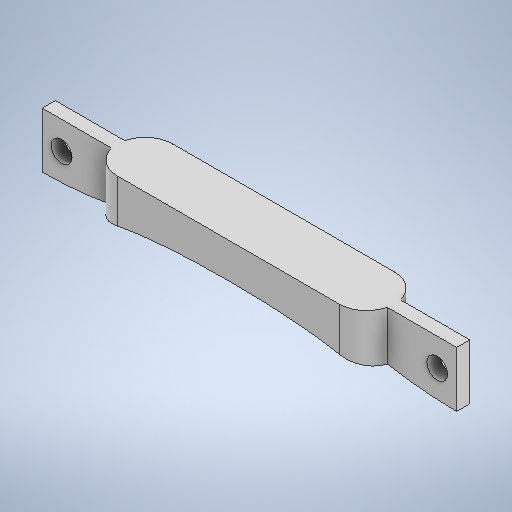
# Autodesk Inventor part: AllFretBars
Saved by Autodesk Inventor 2025.1 (Build 291241000, 241)
## iProperties
Created: 2025-11-05
Part Number: AllFretBars
Material: Generic
Document SubType Name: Modeling
Designer: Juxin
Density: 1 g/cm^3
Appearance: Default
Author: Juxin
Autodesk Inventor part; units mm, degrees
ref_plane "YZ Plane" through (0, 0, 0) normal (1, 0, 0) x (0, 1, 0)
ref_plane "XZ Plane" through (0, 0, 0) normal (0, 1, 0) x (-1, 0, 0)
ref_plane "XY Plane" through (0, 0, 0) normal (0, 0, 1) x (1, 0, 0)
sketch "Sketch1" plane through (0, 0, 0) normal (0, 1, 0) x (-1, 0, 0)
  line L0 (77.4625, -7.85) -> (77.4625, -4.85)
  line L1 (0, 0) -> (17.4625, 0) construction
  line L2 (77.4625, -6.35) -> (77.4625, -4.85)
  line L3 (77.4625, -4.85) -> (61.5875, -4.85)
  line L4 (61.5875, -7.85) -> (77.4625, -7.85)
  line L5 (61.5875, -4.85) -> (61.5875, 0)
  line L6 (61.5875, -7.85) -> (61.5875, -12.7)
  line L7 (61.5875, 0) -> (30, 0)
  line L8 (61.5875, -12.7) -> (30, -12.7)
  line L9 (-17.4625, -7.85) -> (-17.4625, -4.85)
  line L10 (-17.4625, -6.35) -> (-17.4625, -4.85)
  line L11 (-17.4625, -4.85) -> (-1.5875, -4.85)
  line L12 (-1.5875, -7.85) -> (-17.4625, -7.85)
  line L13 (-1.5875, -4.85) -> (-1.5875, 0)
  line L14 (-1.5875, -7.85) -> (-1.5875, -12.7)
  line L15 (-1.5875, 0) -> (30, 0)
  line L16 (-1.5875, -12.7) -> (30, -12.7)
  dimension "d23" = 1.5
  dimension "d24" = 15.875
  dimension "d25" = 3
  dimension "d27" = 63.175
  dimension "d117" = 12.7
  constraints: 34 end point, 2 horizontal, 2 midpoint, 2 perpendicular, 2 point on line
  measures "d23" distance of L0.end L2.start
  measures "d24" distance of L0.end L3.end
  measures "d25" distance of L3.end L4.start
  measures "d27" distance of L13.end L5.end
  measures "d117" distance of L6.end L5.end
extrude "Extrusion1" add sketch "Sketch1" along normal blind 12.7
sketch "Sketch3" plane through (1.5875, 0, -12.7) normal (0, 0, -1) x (-1, 0, 0)
  line L0 (0, 0) -> (63.175, 0) projected
  ellipse E0 centre (31.5875, 0) end of major axis (31.5875, 4.6466) minor radius 31.5875
  point P0 (1.5875, 0)
  constraints: 1 horizontal alignment, 1 midpoint, 2 other
extrude "Extrusion15" cut sketch "Sketch3" against normal blind 20.6375
sketch "Sketch4" plane through (-77.4625, 12.7, -4.85) normal (0, 0, 1) x (1, 0, 0)
  line L0 (15.875, -12.7) -> (15.875, 0) projected
  line L1 (15.875, -6.35) -> (4.445, -6.35)
  circle A0 centre (4.445, -6.35) radius 2.3876
  line L2 (79.05, -12.7) -> (79.05, 0) projected
  line L3 (79.05, -6.35) -> (90.48, -6.35)
  circle A1 centre (90.48, -6.35) radius 2.3876
  point P0 (77.4625, -12.7)
  dimension "d111" = 11.43
  dimension "d112" = 4.7752
  dimension "d113" = 11.43
  dimension "d114" = 4.7752
  constraints: 4 end point, 2 centre point, 2 coincident, 2 horizontal, 2 midpoint
  measures "d111" distance of L1.start L1.end
  measures "d112" diameter of A0
  measures "d113" distance of L3.start L3.end
  measures "d114" diameter of A1
extrude "Extrusion16" cut sketch "Sketch4" against normal blind 58.7375
fillet "Fillet1" radius 92.075 2 edges at (1.5875, 0, -6.35) (-61.5875, 0, -6.35)
fillet "Fillet2" radius 6.35 4 edges at (1.5875, 7.0818, -12.7) (-61.5875, 7.0818, -12.7) (-61.5875, 7.0818, 0) (1.5875, 7.0818, 0)
body "Solid1"
